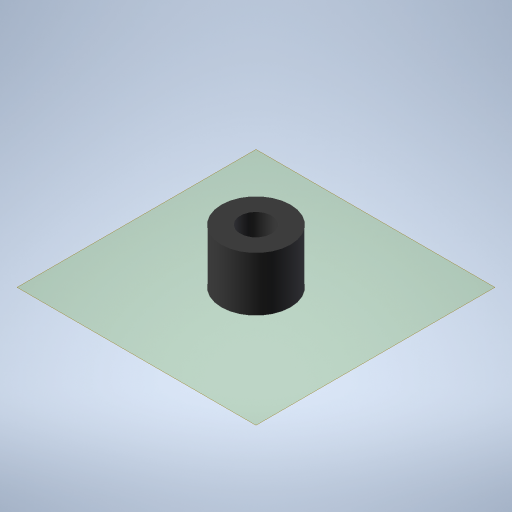
# Autodesk Inventor part: plastic_standoff_10mm
Saved by Autodesk Inventor 2024 (Build 280153000, 153)
## iProperties
Created: 2022-10-07
Part Number: plastic_standoff_10mm
Material: PAEK Plastic
Document SubType Name: Modeling
Designer: raad
Density: 1.32 g/cm^3
Appearance: Default
Author: raad
Autodesk Inventor part; units mm, degrees
ref_plane "YZ Plane" through (0, 0, 0) normal (1, 0, 0) x (0, 1, 0)
ref_plane "XZ Plane" through (0, 0, 0) normal (0, 1, 0) x (-1, 0, 0)
ref_plane "XY Plane" through (0, 0, 0) normal (0, 0, 1) x (1, 0, 0)
ref_plane "Work Plane1" through (0, 0, 0) normal (0, -1, 0) x (1, 0, 0)
sketch "Sketch1" plane through (0, 0, 0) normal (0, -1, 0) x (1, 0, 0)
  circle A0 centre (0, 0) radius 1.4605
  circle A1 centre (0, 0) radius 3.175
  constraints: 2 centre point, 2 coincident
extrude "Extrusion1" add sketch "Sketch1" against normal blind 5
body "Solid3"
